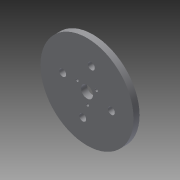
# Autodesk Inventor part: gearSpacerDisc01
Saved by Autodesk Inventor 2013 (Build 170138000, 138)
## iProperties
Created: 2014-07-01
Part Number: gearSpacerDisc01
Material: Generic
Document SubType Name: Modeling
Designer: Nano
Density: 1 g/cm^3
Author: Nano
Autodesk Inventor part; units mm, degrees
ref_plane "YZ Plane" through (0, 0, 0) normal (1, 0, 0) x (0, 1, 0)
ref_plane "XZ Plane" through (0, 0, 0) normal (0, 1, 0) x (-1, 0, 0)
ref_plane "Work Plane1" through (-85.339, 6.6926, 3.8884) normal (0.0215481, -0.1158759, 0.9930299) x (0.9954541, -0.0896829, -0.0320657)
sketch "Sketch1" plane through (-85.339, 6.6926, 3.8884) normal (0.0215481, -0.1158759, 0.9930299) x (0.9954541, -0.0896829, -0.0320657)
  circle A0 centre (85.7068, 3.742) radius 3.175 projected
  circle A1 centre (85.7068, 3.742) radius 24.765
  point P0 (85.676, 0.8558)
  dimension "d0" = 49.53
  constraints: 1 centre point
  measures "d0" diameter of A1
extrude "Extrusion1" add sketch "Sketch1" along normal blind 3.175
sketch "Sketch2" plane through (0.3253, 2.7078, 1.5645) normal (-0.0215481, 0.1158759, -0.9930299) x (-0.9997647, 0, 0.0216942)
  circle A0 centre (12.9454, 2.2936) radius 1.8542
  circle A1 centre (-2.2936, 12.9454) radius 1.8542
  circle A2 centre (-12.9454, -2.2936) radius 1.8542
  circle A3 centre (2.2936, -12.9454) radius 1.8542
  constraints: 4 centre point, 8 other
extrude "Extrusion2" cut sketch "Sketch2" against normal through all
sketch "Sketch3" plane through (0.3937, 2.3399, 4.7174) normal (0.0215481, -0.1158759, 0.9930299) x (0.9997647, 0, -0.0216942)
  circle A0 centre (-5.246, 2.7309) radius 0.762 projected
  circle A1 centre (4.988, 3.1777) radius 0.762 projected
  circle A2 centre (0.258, -5.9086) radius 0.762 projected
extrude "Extrusion3" cut sketch "Sketch3" against normal through all
body "Solid1"
